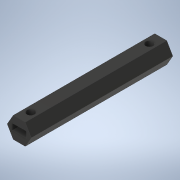
# Autodesk Inventor part: SupportFirstToSecond
Saved by Autodesk Inventor 2020 (Build 240168000, 168)
## iProperties
Created: 2018-12-30
Part Number: SupportFirstToSecond
Material: ABS Plastic
Document SubType Name: Modeling
Designer: Victor Sabino
Density: 1.06 g/cm^3
Appearance: Smooth - White
Mass: 5.01621 g
Surface Area: 28.6628 cm^2
Volume: 4.73227 cm^3
Author: Victor Sabino
Autodesk Inventor part; units mm, degrees
ref_plane "YZ Plane" through (0, 0, 0) normal (1, 0, 0) x (0, 1, 0)
ref_plane "XZ Plane" through (0, 0, 0) normal (0, 1, 0) x (-1, 0, 0)
sketch "Sketch1" plane through (0, 0, 0) normal (0, 0, 1) x (1, 0, 0)
  line L0 (-2.3671, -4.1) -> (-4.7343, 0)
  line L1 (-4.7343, 0) -> (-2.3671, 4.1)
  line L2 (-2.3671, 4.1) -> (2.3671, 4.1)
  line L3 (2.3671, 4.1) -> (4.7343, 0)
  line L4 (4.7343, 0) -> (2.3671, -4.1)
  line L5 (2.3671, -4.1) -> (-2.3671, -4.1)
  point P0 (0, 0)
  point P1 (0, 0)
  dimension "d0" = 4.1
  constraints: 12 end point, 1 coincident, 13 other
  measures "d0" distance from line of L5 point (0, 0)
extrude "Extrusion1" add sketch "Sketch1" against normal blind 55.8
sketch "Sketch2" plane through (4.7343, 0, 0) normal (0.866, 0.5, 0) x (0, 0, -1)
  line L0 (0, 4.7343) -> (0, 0) projected
  line L1 (4.75, 5.1671) -> (7.25, 5.1671)
  line L2 (7.25, 5.1671) -> (7.25, -0.4329)
  line L3 (7.25, -0.4329) -> (4.75, -0.4329)
  line L4 (4.75, -0.4329) -> (4.75, 5.1671)
  line L5 (4.75, 5.1671) -> (7.25, -0.4329) construction
  line L6 (7.25, 5.1671) -> (4.75, -0.4329) construction
  point P0 (0, 2.3671)
  point P1 (6, 2.3671)
  dimension "d3" = 2.5
  dimension "d4" = 5.6
  dimension "d10" = 0
  dimension "d11" = 6
  constraints: 12 end point, 2 midpoint, 2 parallel, 1 horizontal, 1 perpendicular
  measures "d3" distance of L2.end L3.end
  measures "d4" distance of L1.end L2.end
  measures "d10" vertical distance of point (0, 2.367) point (6, 2.367)
  measures "d11" horizontal distance of L0.end point (6, 2.367)
extrude "Extrusion2" [suppressed]
sketch "Sketch3" plane through (0, 0, 0) normal (0, 0, 1) x (1, 0, 0)
  circle A0 centre (0, 0) radius 1.5
  dimension "d7" = 3
  constraints: 1 centre point, 1 coincident
  measures "d7" diameter of A0
extrude "Extrusion3" [suppressed]
ref_plane "Work Plane1" through (0, 0, -27.9) normal (0, 0, -1) x (-1, 0, 0)
mirror "Mirror1" [suppressed]
sketch "Sketch4" plane through (1.5014, 4.1, -7.25) normal (0, 0, 1) x (1, 0, 0)
  line L0 (0, 0) -> (-4.5469, -2.6251) projected
  line L1 (-1.7469, -7.4749) -> (-4.5469, -2.6251) projected
  line L2 (2.8, -4.8497) -> (-1.7469, -7.4749) projected
  line L3 (-4.5469, -2.6251) -> (-4.5469, -5.8583)
  line L4 (-1.7469, -7.4749) -> (-4.5469, -5.8583)
  line L5 (-1.7469, -7.4749) -> (-4.5469, -2.6251)
  point P0 (-1.5014, -4.1)
  dimension "d12" = 120
  dimension "d13" = 120
  constraints: 6 end point, 1 collinear
  measures "d12" angle of L3 L0
  measures "d13" angle of L2 L4
extrude "Extrusion4" [suppressed]
sketch "Sketch5" plane through (-4.7343, 0, -55.8) normal (-0.866, -0.5, 0) x (0, 0, 1)
  line L0 (0, -4.7343) -> (0, 0) projected
  line L1 (4.75, 0.4331) -> (7.25, 0.4331)
  line L2 (7.25, 0.4331) -> (7.25, -5.1669)
  line L3 (7.25, -5.1669) -> (4.75, -5.1669)
  line L4 (4.75, -5.1669) -> (4.75, 0.4331)
  line L5 (4.75, 0.4331) -> (7.25, -5.1669) construction
  line L6 (7.25, 0.4331) -> (4.75, -5.1669) construction
  line L7 (0, -3.8671) -> (0, -0.8671) projected
  line L8 (0, -4.7343) -> (0, 0) projected
  line L9 (0, 0) -> (0, 2.3671) projected
  line L10 (0, 2.3671) -> (0, 0) projected
  line L11 (0, 0) -> (0, -4.7343) projected
  line L12 (0, -4.7343) -> (0, -7.1014) projected
  line L13 (0, -7.1014) -> (0, -4.7343) projected
  line L14 (9.5, -0.8671) -> (9.5, -3.8671) projected
  line L15 (0, -3.8671) -> (0, -0.8671) projected
  line L16 (55.8, -7.1014) -> (0, -7.1014) projected
  line L17 (55.8, 2.3671) -> (0, 2.3671) projected
  point P0 (55.8, -2.3671)
  point P1 (6, -2.3669)
  dimension "d16" = 2.5
  dimension "d17" = 5.6
  dimension "d18" = 6
  dimension "d25" = 1.9345
  constraints: 12 end point, 2 midpoint, 2 parallel, 1 horizontal, 1 perpendicular
  measures "d16" distance of L2.end L3.end
  measures "d17" distance of L1.end L2.end
  measures "d18" distance from line of L0 point (6, -2.367)
  measures "d25" distance between parallel lines of L16 L3
extrude "Extrusion5" [suppressed]
sketch "Sketch6" plane through (-1.5019, -4.1, -42.75) normal (0, 0, -1) x (-1, 0, 0)
  line L0 (-1.7472, 7.4751) -> (-4.5472, 2.6253) projected
  line L1 (-4.5472, 2.6253) -> (-4.5472, 5.8585)
  line L2 (-1.7472, 7.4751) -> (-4.5472, 5.8585)
  line L3 (2.7993, 4.8501) -> (-1.7472, 7.4751) projected
  line L4 (0, 0) -> (-4.5472, 2.6253) projected
  line L5 (-1.7472, 7.4751) -> (-4.5472, 2.6253)
  point P0 (-1.5019, 4.1)
  dimension "d21" = 120
  dimension "d22" = 120
  constraints: 6 end point, 1 perpendicular
  measures "d21" angle of L3 L2
  measures "d22" angle of L4 L1
extrude "Extrusion6" [suppressed]
sketch "Sketch8" plane through (0, 0, -55.8) normal (0, 0, -1) x (-1, 0, 0)
  line L0 (-2.8, 1.25) -> (2.8, 1.25)
  line L1 (2.8, 1.25) -> (2.8, -1.25)
  line L2 (2.8, -1.25) -> (-2.8, -1.25)
  line L3 (-2.8, -1.25) -> (-2.8, 1.25)
  line L4 (-2.8, 1.25) -> (2.8, -1.25) construction
  line L5 (2.8, 1.25) -> (-2.8, -1.25) construction
  point P0 (0, 0)
  dimension "d32" = 5.6
  dimension "d33" = 2.5
  dimension "d46" = 1.25
  dimension "d47" = 2.8
  constraints: 12 end point, 2 parallel, 1 horizontal, 1 perpendicular
  measures "d32" distance of L1.end L2.end
  measures "d33" distance of L0.end L1.end
  measures "d46" distance from line of point (0, 0) L0
  measures "d47" distance from line of L3 point (0, 0)
extrude "Extrusion8" cut sketch "Sketch8" against normal blind 6.5
sketch "Sketch9" plane through (-2.3671, 4.1, 0) normal (0, 1, 0) x (1, 0, 0)
  line L0 (4.7343, 0) -> (4.7343, 55.8) projected
  line L1 (0, 55.8) -> (4.7343, 55.8) projected
  line L2 (0, 0) -> (0, 55.8) projected
  line L3 (0, 0) -> (4.7343, 0) projected
  line L4 (5.1671, 55.8) -> (-0.4329, 55.8) projected
  line L5 (2.3671, 55.8) -> (2.3671, 0) construction
  line L6 (2.3671, 55.8) -> (58.1671, 55.8) construction
  circle A0 centre (2.3671, 51.3) radius 1.5
  dimension "d36" = 90
  dimension "d37" = 3
  dimension "d38" = 0
  dimension "d39" = 4.5
  constraints: 4 end point, 1 centre point, 1 horizontal, 1 midpoint, 1 perpendicular, 1 vertical
  measures "d36" angle of L5 L6
  measures "d37" diameter of A0
  measures "d38" distance from line of L5 A0.centre
  measures "d39" distance of L5.start A0.centre
extrude "Extrusion9" cut sketch "Sketch9" against normal up to surface (8.2 mm away) contours A0
sketch "Sketch10" plane through (-2.8, 1.25, -55.8) normal (0, -1, 0) x (1, 0, 0)
  circle A0 centre (2.8, 4.5) radius 1.5 projected
  line L0 (5.6, 0) -> (0, 0) projected
  line L1 (5.6, 0) -> (5.6, 6.5) projected
  line L2 (5.6, 6.5) -> (0, 6.5) projected
  line L3 (0, 0) -> (0, 6.5) projected
  line L4 (0, 6.5) -> (2.8, 8.1166)
  line L5 (0, 6.5) -> (3.9156, 6.5) construction
  line L6 (5.6, 6.5) -> (2.8, 8.1166)
  line L7 (5.6, 6.5) -> (8.8332, 6.5) construction
  line L8 (5.6, 6.5) -> (0, 6.5)
  point P0 (2.8, 55.8)
  dimension "d42" = 30
  dimension "d43" = 150
  constraints: 10 end point, 2 horizontal, 1 collinear, 1 equal length
  measures "d42" angle of L5 L4
  measures "d43" angle of L7 L6
extrude "Extrusion10" cut sketch "Sketch10" along normal blind 2.5 contours L2 L4 L6
mirror "Mirror3" about plane through (0, 0, -27.9) normal (0, 0, -1) of "Extrusion8", "Extrusion9", "Extrusion10"
body "Solid1"
